Autodesk Fusion 360 part; units mm, degrees
(part 2 of 2)
extrude "Extrude4" add sketch "Sketch4" along normal blind 4 contours L42 L43 L44 A16 L45 L46 L47 L76 L77 L78 | L0 L1 L2 A2 L3 L4 L5 L81 L82 L83 | A16 L74 A22 L75 | A2 L79 A23 L80 | L36 L37 L38 A14 L39 L40 L41 L71 L72 L73 | L6 L7 L8 A4 L9 L10 L11 L86 L87 L88 | A14 L69 A21 L70 | A4 L84 A24 L85 | L30 L31 L32 A12 L33 L34 L35 L66 L67 L68 | L12 L13 L14 A6 L15 L16 L17 L50 L51 L52 L53 | A12 L64 A20 L65 | A6 L48 L49 A17 | L24 L25 L26 A10 L27 L28 L29 L61 L62 L63 | L18 L19 L20 A8 L21 L22 L23 L56 L57 L58 | A10 L59 A19 L60 | A8 L54 A18 L55 bodies 1 2
sketch "Sketch5" plane through (0, 0, 2) normal (0, 0, 1) x (-1, 0, 0)
  line L0 (9.1045, -28.6592) -> (7.2341, -23.9305)
  arc A0 (-6.6853, -24.0896) -> (7.2341, -23.9305) centre (0, 0) ccw
  line L1 (-6.6853, -24.0896) -> (-8.26, -28.886)
  arc A1 (-13.8273, -26.703) -> (-8.26, -28.886) centre (-11.0437, -27.7945) ccw
  line L2 (-13.8273, -26.703) -> (-11.8061, -22.0367)
  arc A2 (-21.7611, -12.3067) -> (-11.8061, -22.0367) centre (0, 0) ccw
  line L3 (-21.7611, -12.3067) -> (-26.2662, -14.5848)
  arc A3 (-28.6592, -9.1045) -> (-26.2662, -14.5848) centre (-27.4627, -11.8446) ccw
  line L4 (-28.6592, -9.1045) -> (-23.9305, -7.2341)
  arc A4 (-24.0896, 6.6853) -> (-23.9305, -7.2341) centre (0, 0) ccw
  line L5 (-24.0896, 6.6853) -> (-28.886, 8.26)
  arc A5 (-26.703, 13.8273) -> (-28.886, 8.26) centre (-27.7945, 11.0437) ccw
  line L6 (-26.703, 13.8273) -> (-22.0367, 11.8061)
  arc A6 (-12.3067, 21.7611) -> (-22.0367, 11.8061) centre (0, 0) ccw
  line L7 (-12.3067, 21.7611) -> (-14.5848, 26.2662)
  arc A7 (-9.1045, 28.6592) -> (-14.5848, 26.2662) centre (-11.8446, 27.4627) ccw
  line L8 (-9.1045, 28.6592) -> (-7.2341, 23.9305)
  arc A8 (6.6853, 24.0896) -> (-7.2341, 23.9305) centre (0, 0) ccw
  line L9 (6.6853, 24.0896) -> (8.26, 28.886)
  arc A9 (13.8273, 26.703) -> (8.26, 28.886) centre (11.0437, 27.7945) ccw
  line L10 (13.8273, 26.703) -> (11.8061, 22.0367)
  arc A10 (21.7611, 12.3067) -> (11.8061, 22.0367) centre (0, 0) ccw
  line L11 (21.7611, 12.3067) -> (26.2662, 14.5848)
  arc A11 (28.6592, 9.1045) -> (26.2662, 14.5848) centre (27.4627, 11.8446) ccw
  line L12 (28.6592, 9.1045) -> (23.9305, 7.2341)
  arc A12 (24.0896, -6.6853) -> (23.9305, 7.2341) centre (0, 0) ccw
  line L13 (24.0896, -6.6853) -> (28.886, -8.26)
  arc A13 (26.703, -13.8273) -> (28.886, -8.26) centre (27.7945, -11.0437) ccw
  line L14 (26.703, -13.8273) -> (22.0367, -11.8061)
  arc A14 (12.3067, -21.7611) -> (22.0367, -11.8061) centre (0, 0) ccw
  line L15 (12.3067, -21.7611) -> (14.5848, -26.2662)
  arc A15 (9.1045, -28.6592) -> (14.5848, -26.2662) centre (11.8446, -27.4627) ccw
  circle A16 centre (0, 0) radius 36.6
  circle A17 centre (0, -32) radius 1.6
  circle A18 centre (32, 0) radius 1.6
  circle A19 centre (0, 32) radius 1.6
  circle A20 centre (-32, 0) radius 1.6
  dimension "d33" = 3.2
  dimension "d34" = 32
  dimension "d36" = 360
  constraint vertical A0.centre A17.centre
  measures "d33" diameter of A17
  measures "d34" vertical distance of A0.centre A17.centre
extrude "Extrude5" cut sketch "Sketch5" against normal through all contours A17 | A18 | A19 | A20 bodies 1
